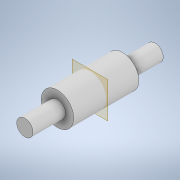
# Autodesk Inventor part: WellenSchiffsschraube2
Saved by Autodesk Inventor 2021 (Build 250183000, 183)
## iProperties
Created: 2021-01-12
Part Number: WellenSchiffsschraube2
Material: Generisch
Document SubType Name: Modeling
Designer: casa2
Density: 1 g/cm^3
Appearance: Vorgabe
Author: casa2
Autodesk Inventor part; units mm, degrees
ref_plane "YZ Plane" through (0, 0, 0) normal (1, 0, 0) x (0, 1, 0)
ref_plane "XZ Plane" through (0, 0, 0) normal (0, 1, 0) x (-1, 0, 0)
sketch "Skizze1" plane through (0, 0, 0) normal (0, 0, 1) x (1, 0, 0)
  circle A0 centre (0, 0) radius 5
  dimension "d0" = 10
  constraints: 1 centre point, 1 coincident
  measures "d0" diameter of A0
extrude "Extrusion1" add sketch "Skizze1" along normal blind 20
sketch "Skizze6" plane through (0, 0, 0) normal (0, 0, -1) x (-1, 0, 0)
  circle A0 centre (0, 0) radius 5 projected
  circle A1 centre (0, 0) radius 2.5
  dimension "d25" = 5
  constraints: 1 centre point, 1 coincident
  measures "d25" diameter of A1
extrude "Extrusion6" add sketch "Skizze6" along normal blind 10 contours A1
ref_plane "Arbeitsebene3" through (0, 0, 10) normal (0, 0, 1) x (1, 0, 0)
mirror "Spiegeln2" about plane through (0, 0, 10) normal (0, 0, 1) of "Extrusion6"
equation "\"d0\" = Durchmesser3"
equation "\"Durchmesser1\" = 15"
equation "\"Größe1\" = 7"
equation "\"Durchmesser2\" = 3"
equation "\"Durchmesser3\" = 10"
equation "\"Größe3\" = 3"
equation "\"Größe4\" = 15"
